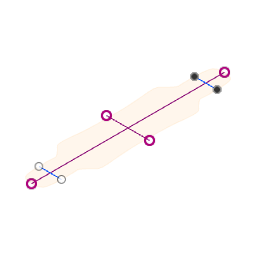
LongBoard v1 (Autodesk Fusion 360 design; units mm, degrees)
Autodesk Fusion 360 part; units mm, degrees
sketch "Sketch1" plane through (0, 0, 0) normal (0, 1, 0) x (1, 0, 0)
  line L0 (1.5, -63) -> (1.5, 40)
  line L1 (-10, -11.5) -> (13, -11.5)
  spline S0 degree 5 poles (1.5, 39.8994) (1.4399, 39.8994) (1.3198, 39.8994) (1.1397, 39.8994) (0.8995, 39.8994) (0.5992, 39.8994) (0.359, 39.8994) (0.1788, 39.8994) (0.0587, 39.8994) (-0.0013, 39.8994) knots 0 0 0 0 0 0 0.2 0.4 0.6 0.8 1 1 1 1 1 1
  spline S1 degree 5 poles (-0.0013, 39.8994) (-0.0218, 39.8979) (-0.0631, 39.8948) (-0.1256, 39.8901) (-0.2101, 39.8836) (-0.3178, 39.8751) (-0.4274, 39.866) (-0.539, 39.8561) (-0.6523, 39.8451) (-0.7672, 39.8322) (-0.8833, 39.8166) (-1.0002, 39.7977) (-1.1173, 39.7746) (-1.2334, 39.7472) (-1.3473, 39.7155) (-1.457, 39.6802) (-1.5606, 39.6428) (-1.6561, 39.6046) (-1.7423, 39.5672) (-1.8188, 39.5315) (-1.887, 39.4978) (-1.9498, 39.4653) (-2.0108, 39.4326) (-2.0739, 39.398) (-2.1421, 39.3599) (-2.2168, 39.3165) (-2.2984, 39.2666) (-2.3861, 39.2095) (-2.4785, 39.1451) (-2.5733, 39.074) (-2.6681, 38.9982) (-2.7601, 38.9197) (-2.847, 38.8412) (-2.9267, 38.765) (-2.9978, 38.693) (-3.0602, 38.6264) (-3.1145, 38.5652) (-3.1625, 38.5087) (-3.2058, 38.4556) (-3.2464, 38.4044) (-3.2854, 38.3535) (-3.3238, 38.3017) (-3.3617, 38.2481) (-3.399, 38.1932) (-3.4348, 38.1384) (-3.4682, 38.0857) (-3.4986, 38.0364) (-3.526, 37.9902) (-3.5515, 37.9451) (-3.5761, 37.8985) (-3.6006, 37.849) (-3.6247, 37.7981) (-3.6475, 37.7483) (-3.6682, 37.7019) (-3.6867, 37.6585) (-3.7041, 37.6146) (-3.7216, 37.5664) (-3.7401, 37.5116) (-3.7593, 37.4514) (-3.7786, 37.3886) (-3.7971, 37.3266) (-3.8143, 37.2668) (-3.8302, 37.2087) (-3.8451, 37.1506) (-3.8597, 37.0905) (-3.8743, 37.0273) (-3.8893, 36.9608) (-3.9052, 36.8908) (-3.922, 36.8176) (-3.9395, 36.7407) (-3.9576, 36.6596) (-3.9757, 36.5739) (-3.9934, 36.4839) (-4.0103, 36.3909) (-4.0261, 36.2973) (-4.0406, 36.2061) (-4.0536, 36.1202) (-4.0654, 36.0413) (-4.0759, 35.9695) (-4.0855, 35.9031) (-4.0946, 35.8392) (-4.1035, 35.775) (-4.1124, 35.7085) (-4.1217, 35.639) (-4.1314, 35.5666) (-4.1416, 35.4919) (-4.152, 35.4162) (-4.1625, 35.3404) (-4.1727, 35.2657) (-4.1824, 35.1926) (-4.1915, 35.1209) (-4.2002, 35.0493) (-4.2087, 34.9764) (-4.2174, 34.9005) (-4.2265, 34.8206) (-4.2359, 34.7364) (-4.2456, 34.6486) (-4.2552, 34.5584) (-4.2646, 34.4672) (-4.2736, 34.3769) (-4.2821, 34.2889) (-4.2901, 34.2046) (-4.2977, 34.1248) (-4.3048, 34.0496) (-4.3115, 33.9782) (-4.318, 33.9088) (-4.3244, 33.8391) (-4.3307, 33.7658) (-4.3372, 33.6856) (-4.3442, 33.5945) (-4.3518, 33.4891) (-4.3603, 33.3661) (-4.3699, 33.2229) (-4.3806, 33.0582) (-4.3925, 32.8718) (-4.4053, 32.6647) (-4.4189, 32.4387) (-4.433, 32.1966) (-4.4474, 31.9415) (-4.4617, 31.677) (-4.4756, 31.4069) (-4.4888, 31.1352) (-4.5011, 30.8654) (-4.5122, 30.6012) (-4.522, 30.3455) (-4.5305, 30.1006) (-4.5377, 29.8683) (-4.5436, 29.6498) (-4.5484, 29.4457) (-4.5522, 29.2561) (-4.5552, 29.0807) (-4.5576, 28.9186) (-4.5595, 28.7685) (-4.5611, 28.6286) (-4.5624, 28.4967) (-4.5636, 28.3702) (-4.5646, 28.2466) (-4.5654, 28.1229) (-4.5661, 27.9966) (-4.5666, 27.8653) (-4.5669, 27.7268) (-4.567, 27.5796) (-4.5669, 27.4226) (-4.5665, 27.2548) (-4.5659, 27.0757) (-4.5651, 26.8851) (-4.5642, 26.7231) (-4.5634, 26.5963) (-4.5628, 26.5094) (-4.5625, 26.4653) knots 0 0 0 0 0 0 0.00689655 0.0137931 0.02068966 0.02758621 0.03448276 0.04137931 0.04827586 0.05517241 0.06206897 0.06896552 0.07586207 0.08275862 0.08965517 0.09655172 0.10344828 0.11034483 0.11724138 0.12413793 0.13103448 0.13793103 0.14482759 0.15172414 0.15862069 0.16551724 0.17241379 0.17931034 0.1862069 0.19310345 0.2 0.20689655 0.2137931 0.22068966 0.22758621 0.23448276 0.24137931 0.24827586 0.25517241 0.26206897 0.26896552 0.27586207 0.28275862 0.28965517 0.29655172 0.30344828 0.31034483 0.31724138 0.32413793 0.33103448 0.33793103 0.34482759 0.35172414 0.35862069 0.36551724 0.37241379 0.37931034 0.3862069 0.39310345 0.4 0.40689655 0.4137931 0.42068966 0.42758621 0.43448276 0.44137931 0.44827586 0.45517241 0.46206897 0.46896552 0.47586207 0.48275862 0.48965517 0.49655172 0.50344828 0.51034483 0.51724138 0.52413793 0.53103448 0.53793103 0.54482759 0.55172414 0.55862069 0.56551724 0.57241379 0.57931034 0.5862069 0.59310345 0.6 0.60689655 0.6137931 0.62068966 0.62758621 0.63448276 0.64137931 0.64827586 0.65517241 0.66206897 0.66896552 0.67586207 0.68275862 0.68965517 0.69655172 0.70344828 0.71034483 0.71724138 0.72413793 0.73103448 0.73793103 0.74482759 0.75172414 0.75862069 0.76551724 0.77241379 0.77931034 0.7862069 0.79310345 0.8 0.80689655 0.8137931 0.82068966 0.82758621 0.83448276 0.84137931 0.84827586 0.85517241 0.86206897 0.86896552 0.87586207 0.88275862 0.88965517 0.89655172 0.90344828 0.91034483 0.91724138 0.92413793 0.93103448 0.93793103 0.94482759 0.95172414 0.95862069 0.96551724 0.97241379 0.97931034 0.9862069 0.99310345 1 1 1 1 1 1
  spline S2 degree 5 poles (-4.5625, 26.4653) (-4.5655, 26.3307) (-4.57, 26.0496) (-4.572, 25.5928) (-4.5661, 24.9124) (-4.5379, 23.9635) (-4.4825, 22.9635) (-4.3594, 22.0422) (-4.344, 21.226) (-4.6467, 20.4795) (-5.3052, 19.6439) (-6.1392, 18.6182) (-7.0385, 17.5852) (-7.8877, 16.7191) (-8.6091, 16.1406) (-9.1643, 15.5973) (-9.5444, 14.8768) (-9.7555, 13.8923) (-9.8172, 12.6021) (-9.7558, 10.9978) (-9.602, 9.0799) (-9.389, 6.8619) (-9.151, 4.3636) (-8.9215, 1.6101) (-8.732, -1.3722) (-8.61, -4.5579) (-8.5838, -7.2519) (-8.6109, -9.3475) (-8.6505, -10.7771) (-8.6757, -11.5) knots 0 0 0 0 0 0 0.04 0.08 0.12 0.16 0.2 0.24 0.28 0.32 0.36 0.4 0.44 0.48 0.52 0.56 0.6 0.64 0.68 0.72 0.76 0.8 0.84 0.88 0.92 0.96 1 1 1 1 1 1
  line L2 (-5.8, 18.6) -> (-11, 14)
  line L3 (-2.8, 23.5) -> (-6.8, 17.2)
  line L4 (-4.8152, 28.0337) -> (-4.1848, 18.7663)
  line L5 (-8.4763, -5.7777) -> (-8.8751, -17.2223)
  spline S3 degree 5 poles (-4.5625, -49.4653) (-4.5655, -49.3307) (-4.57, -49.0496) (-4.572, -48.5928) (-4.5661, -47.9124) (-4.5379, -46.9635) (-4.4825, -45.9635) (-4.3594, -45.0422) (-4.344, -44.226) (-4.6467, -43.4795) (-5.3052, -42.6439) (-6.1392, -41.6182) (-7.0385, -40.5852) (-7.8877, -39.7191) (-8.6091, -39.1406) (-9.1643, -38.5973) (-9.5444, -37.8768) (-9.7555, -36.8923) (-9.8172, -35.6021) (-9.7558, -33.9978) (-9.602, -32.0799) (-9.389, -29.8619) (-9.151, -27.3636) (-8.9215, -24.6101) (-8.732, -21.6278) (-8.61, -18.4421) (-8.5838, -15.7481) (-8.6109, -13.6525) (-8.6505, -12.2229) (-8.6757, -11.5) knots 0 0 0 0 0 0 0.04 0.08 0.12 0.16 0.2 0.24 0.28 0.32 0.36 0.4 0.44 0.48 0.52 0.56 0.6 0.64 0.68 0.72 0.76 0.8 0.84 0.88 0.92 0.96 1 1 1 1 1 1
  line L6 (-4.4911, 29.6841) -> (-4.634, 23.2466)
  line L7 (-4.4911, -52.6841) -> (-4.634, -46.2466)
  line L8 (-4.8152, -51.0337) -> (-4.1848, -41.7663)
  line L9 (-2.8, -46.5) -> (-6.8, -40.2)
  line L10 (-5.8, -41.6) -> (-11, -37)
  line L11 (-8.4763, -17.2223) -> (-8.8751, -5.7777)
  spline S4 degree 5 poles (-0.0013, -62.8994) (-0.0218, -62.8979) (-0.0631, -62.8948) (-0.1256, -62.8901) (-0.2101, -62.8836) (-0.3178, -62.8751) (-0.4274, -62.866) (-0.539, -62.8561) (-0.6523, -62.8451) (-0.7672, -62.8322) (-0.8833, -62.8166) (-1.0002, -62.7977) (-1.1173, -62.7746) (-1.2334, -62.7472) (-1.3473, -62.7155) (-1.457, -62.6802) (-1.5606, -62.6428) (-1.6561, -62.6046) (-1.7423, -62.5672) (-1.8188, -62.5315) (-1.887, -62.4978) (-1.9498, -62.4653) (-2.0108, -62.4326) (-2.0739, -62.398) (-2.1421, -62.3599) (-2.2168, -62.3165) (-2.2984, -62.2666) (-2.3861, -62.2095) (-2.4785, -62.1451) (-2.5733, -62.074) (-2.6681, -61.9982) (-2.7601, -61.9197) (-2.847, -61.8412) (-2.9267, -61.765) (-2.9978, -61.693) (-3.0602, -61.6264) (-3.1145, -61.5652) (-3.1625, -61.5087) (-3.2058, -61.4556) (-3.2464, -61.4044) (-3.2854, -61.3535) (-3.3238, -61.3017) (-3.3617, -61.2481) (-3.399, -61.1932) (-3.4348, -61.1384) (-3.4682, -61.0857) (-3.4986, -61.0364) (-3.526, -60.9902) (-3.5515, -60.9451) (-3.5761, -60.8985) (-3.6006, -60.849) (-3.6247, -60.7981) (-3.6475, -60.7483) (-3.6682, -60.7019) (-3.6867, -60.6585) (-3.7041, -60.6146) (-3.7216, -60.5664) (-3.7401, -60.5116) (-3.7593, -60.4514) (-3.7786, -60.3886) (-3.7971, -60.3266) (-3.8143, -60.2668) (-3.8302, -60.2087) (-3.8451, -60.1506) (-3.8597, -60.0905) (-3.8743, -60.0273) (-3.8893, -59.9608) (-3.9052, -59.8908) (-3.922, -59.8176) (-3.9395, -59.7407) (-3.9576, -59.6596) (-3.9757, -59.5739) (-3.9934, -59.4839) (-4.0103, -59.3909) (-4.0261, -59.2973) (-4.0406, -59.2061) (-4.0536, -59.1202) (-4.0654, -59.0413) (-4.0759, -58.9695) (-4.0855, -58.9031) (-4.0946, -58.8392) (-4.1035, -58.775) (-4.1124, -58.7085) (-4.1217, -58.639) (-4.1314, -58.5666) (-4.1416, -58.4919) (-4.152, -58.4162) (-4.1625, -58.3404) (-4.1727, -58.2657) (-4.1824, -58.1926) (-4.1915, -58.1209) (-4.2002, -58.0493) (-4.2087, -57.9764) (-4.2174, -57.9005) (-4.2265, -57.8206) (-4.2359, -57.7364) (-4.2456, -57.6486) (-4.2552, -57.5584) (-4.2646, -57.4672) (-4.2736, -57.3769) (-4.2821, -57.2889) (-4.2901, -57.2046) (-4.2977, -57.1248) (-4.3048, -57.0496) (-4.3115, -56.9782) (-4.318, -56.9088) (-4.3244, -56.8391) (-4.3307, -56.7658) (-4.3372, -56.6856) (-4.3442, -56.5945) (-4.3518, -56.4891) (-4.3603, -56.3661) (-4.3699, -56.2229) (-4.3806, -56.0582) (-4.3925, -55.8718) (-4.4053, -55.6647) (-4.4189, -55.4387) (-4.433, -55.1966) (-4.4474, -54.9415) (-4.4617, -54.677) (-4.4756, -54.4069) (-4.4888, -54.1352) (-4.5011, -53.8654) (-4.5122, -53.6012) (-4.522, -53.3455) (-4.5305, -53.1006) (-4.5377, -52.8683) (-4.5436, -52.6498) (-4.5484, -52.4457) (-4.5522, -52.2561) (-4.5552, -52.0807) (-4.5576, -51.9186) (-4.5595, -51.7685) (-4.5611, -51.6286) (-4.5624, -51.4967) (-4.5636, -51.3702) (-4.5646, -51.2466) (-4.5654, -51.1229) (-4.5661, -50.9966) (-4.5666, -50.8653) (-4.5669, -50.7268) (-4.567, -50.5796) (-4.5669, -50.4226) (-4.5665, -50.2548) (-4.5659, -50.0757) (-4.5651, -49.8851) (-4.5642, -49.7231) (-4.5634, -49.5963) (-4.5628, -49.5094) (-4.5625, -49.4653) knots 0 0 0 0 0 0 0.00689655 0.0137931 0.02068966 0.02758621 0.03448276 0.04137931 0.04827586 0.05517241 0.06206897 0.06896552 0.07586207 0.08275862 0.08965517 0.09655172 0.10344828 0.11034483 0.11724138 0.12413793 0.13103448 0.13793103 0.14482759 0.15172414 0.15862069 0.16551724 0.17241379 0.17931034 0.1862069 0.19310345 0.2 0.20689655 0.2137931 0.22068966 0.22758621 0.23448276 0.24137931 0.24827586 0.25517241 0.26206897 0.26896552 0.27586207 0.28275862 0.28965517 0.29655172 0.30344828 0.31034483 0.31724138 0.32413793 0.33103448 0.33793103 0.34482759 0.35172414 0.35862069 0.36551724 0.37241379 0.37931034 0.3862069 0.39310345 0.4 0.40689655 0.4137931 0.42068966 0.42758621 0.43448276 0.44137931 0.44827586 0.45517241 0.46206897 0.46896552 0.47586207 0.48275862 0.48965517 0.49655172 0.50344828 0.51034483 0.51724138 0.52413793 0.53103448 0.53793103 0.54482759 0.55172414 0.55862069 0.56551724 0.57241379 0.57931034 0.5862069 0.59310345 0.6 0.60689655 0.6137931 0.62068966 0.62758621 0.63448276 0.64137931 0.64827586 0.65517241 0.66206897 0.66896552 0.67586207 0.68275862 0.68965517 0.69655172 0.70344828 0.71034483 0.71724138 0.72413793 0.73103448 0.73793103 0.74482759 0.75172414 0.75862069 0.76551724 0.77241379 0.77931034 0.7862069 0.79310345 0.8 0.80689655 0.8137931 0.82068966 0.82758621 0.83448276 0.84137931 0.84827586 0.85517241 0.86206897 0.86896552 0.87586207 0.88275862 0.88965517 0.89655172 0.90344828 0.91034483 0.91724138 0.92413793 0.93103448 0.93793103 0.94482759 0.95172414 0.95862069 0.96551724 0.97241379 0.97931034 0.9862069 0.99310345 1 1 1 1 1 1
  line L12 (1.5328, 40.0122) -> (-1.5354, 39.7866)
  line L13 (-4.5763, 28.5249) -> (-4.5488, 24.4057)
  line L14 (1.5328, -63.0122) -> (-1.5354, -62.7866)
  line L15 (-4.5763, -51.5249) -> (-4.5488, -47.4057)
  spline S5 degree 5 poles (1.5, -62.8994) (1.4399, -62.8994) (1.3198, -62.8994) (1.1397, -62.8994) (0.8995, -62.8994) (0.5992, -62.8994) (0.359, -62.8994) (0.1788, -62.8994) (0.0587, -62.8994) (-0.0013, -62.8994) knots 0 0 0 0 0 0 0.2 0.4 0.6 0.8 1 1 1 1 1 1
  line L16 (1.6531, 39.8994) -> (1.3469, 39.8994)
  line L17 (0.1518, 39.8994) -> (-0.1544, 39.8994)
  line L18 (1.6531, -62.8994) -> (1.3469, -62.8994)
  line L19 (0.1518, -62.8994) -> (-0.1544, -62.8994)
  spline S6 degree 5 poles (7.5625, 26.4653) (7.5655, 26.3307) (7.57, 26.0496) (7.572, 25.5928) (7.5661, 24.9124) (7.5379, 23.9635) (7.4825, 22.9635) (7.3594, 22.0422) (7.344, 21.226) (7.6467, 20.4795) (8.3052, 19.6439) (9.1392, 18.6182) (10.0385, 17.5852) (10.8877, 16.7191) (11.6091, 16.1406) (12.1643, 15.5973) (12.5444, 14.8768) (12.7555, 13.8923) (12.8172, 12.6021) (12.7558, 10.9978) (12.602, 9.0799) (12.389, 6.8619) (12.151, 4.3636) (11.9215, 1.6101) (11.732, -1.3722) (11.61, -4.5579) (11.5838, -7.2519) (11.6109, -9.3475) (11.6505, -10.7771) (11.6757, -11.5) knots 0 0 0 0 0 0 0.04 0.08 0.12 0.16 0.2 0.24 0.28 0.32 0.36 0.4 0.44 0.48 0.52 0.56 0.6 0.64 0.68 0.72 0.76 0.8 0.84 0.88 0.92 0.96 1 1 1 1 1 1
  line L20 (7.4911, 29.6841) -> (7.634, 23.2466)
  line L21 (7.8152, 28.0337) -> (7.1848, 18.7663)
  line L22 (5.8, 23.5) -> (9.8, 17.2)
  line L23 (8.8, 18.6) -> (14, 14)
  line L24 (11.4763, -5.7777) -> (11.8751, -17.2223)
  spline S7 degree 5 poles (7.5625, -49.4653) (7.5655, -49.3307) (7.57, -49.0496) (7.572, -48.5928) (7.5661, -47.9124) (7.5379, -46.9635) (7.4825, -45.9635) (7.3594, -45.0422) (7.344, -44.226) (7.6467, -43.4795) (8.3052, -42.6439) (9.1392, -41.6182) (10.0385, -40.5852) (10.8877, -39.7191) (11.6091, -39.1406) (12.1643, -38.5973) (12.5444, -37.8768) (12.7555, -36.8923) (12.8172, -35.6021) (12.7558, -33.9978) (12.602, -32.0799) (12.389, -29.8619) (12.151, -27.3636) (11.9215, -24.6101) (11.732, -21.6278) (11.61, -18.4421) (11.5838, -15.7481) (11.6109, -13.6525) (11.6505, -12.2229) (11.6757, -11.5) knots 0 0 0 0 0 0 0.04 0.08 0.12 0.16 0.2 0.24 0.28 0.32 0.36 0.4 0.44 0.48 0.52 0.56 0.6 0.64 0.68 0.72 0.76 0.8 0.84 0.88 0.92 0.96 1 1 1 1 1 1
  line L25 (7.4911, -52.6841) -> (7.634, -46.2466)
  line L26 (7.8152, -51.0337) -> (7.1848, -41.7663)
  line L27 (5.8, -46.5) -> (9.8, -40.2)
  line L28 (8.8, -41.6) -> (14, -37)
  line L29 (11.4763, -17.2223) -> (11.8751, -5.7777)
  spline S8 degree 5 poles (3.0013, 39.8994) (3.0218, 39.8979) (3.0631, 39.8948) (3.1256, 39.8901) (3.2101, 39.8836) (3.3178, 39.8751) (3.4274, 39.866) (3.539, 39.8561) (3.6523, 39.8451) (3.7672, 39.8322) (3.8833, 39.8166) (4.0002, 39.7977) (4.1173, 39.7746) (4.2334, 39.7472) (4.3473, 39.7155) (4.457, 39.6802) (4.5606, 39.6428) (4.6561, 39.6046) (4.7423, 39.5672) (4.8188, 39.5315) (4.887, 39.4978) (4.9498, 39.4653) (5.0108, 39.4326) (5.0739, 39.398) (5.1421, 39.3599) (5.2168, 39.3165) (5.2984, 39.2666) (5.3861, 39.2095) (5.4785, 39.1451) (5.5733, 39.074) (5.6681, 38.9982) (5.7601, 38.9197) (5.847, 38.8412) (5.9267, 38.765) (5.9978, 38.693) (6.0602, 38.6264) (6.1145, 38.5652) (6.1625, 38.5087) (6.2058, 38.4556) (6.2464, 38.4044) (6.2854, 38.3535) (6.3238, 38.3017) (6.3617, 38.2481) (6.399, 38.1932) (6.4348, 38.1384) (6.4682, 38.0857) (6.4986, 38.0364) (6.526, 37.9902) (6.5515, 37.9451) (6.5761, 37.8985) (6.6006, 37.849) (6.6247, 37.7981) (6.6475, 37.7483) (6.6682, 37.7019) (6.6867, 37.6585) (6.7041, 37.6146) (6.7216, 37.5664) (6.7401, 37.5116) (6.7593, 37.4514) (6.7786, 37.3886) (6.7971, 37.3266) (6.8143, 37.2668) (6.8302, 37.2087) (6.8451, 37.1506) (6.8597, 37.0905) (6.8743, 37.0273) (6.8893, 36.9608) (6.9052, 36.8908) (6.922, 36.8176) (6.9395, 36.7407) (6.9576, 36.6596) (6.9757, 36.5739) (6.9934, 36.4839) (7.0103, 36.3909) (7.0261, 36.2973) (7.0406, 36.2061) (7.0536, 36.1202) (7.0654, 36.0413) (7.0759, 35.9695) (7.0855, 35.9031) (7.0946, 35.8392) (7.1035, 35.775) (7.1124, 35.7085) (7.1217, 35.639) (7.1314, 35.5666) (7.1416, 35.4919) (7.152, 35.4162) (7.1625, 35.3404) (7.1727, 35.2657) (7.1824, 35.1926) (7.1915, 35.1209) (7.2002, 35.0493) (7.2087, 34.9764) (7.2174, 34.9005) (7.2265, 34.8206) (7.2359, 34.7364) (7.2456, 34.6486) (7.2552, 34.5584) (7.2646, 34.4672) (7.2736, 34.3769) (7.2821, 34.2889) (7.2901, 34.2046) (7.2977, 34.1248) (7.3048, 34.0496) (7.3115, 33.9782) (7.318, 33.9088) (7.3244, 33.8391) (7.3307, 33.7658) (7.3372, 33.6856) (7.3442, 33.5945) (7.3518, 33.4891) (7.3603, 33.3661) (7.3699, 33.2229) (7.3806, 33.0582) (7.3925, 32.8718) (7.4053, 32.6647) (7.4189, 32.4387) (7.433, 32.1966) (7.4474, 31.9415) (7.4617, 31.677) (7.4756, 31.4069) (7.4888, 31.1352) (7.5011, 30.8654) (7.5122, 30.6012) (7.522, 30.3455) (7.5305, 30.1006) (7.5377, 29.8683) (7.5436, 29.6498) (7.5484, 29.4457) (7.5522, 29.2561) (7.5552, 29.0807) (7.5576, 28.9186) (7.5595, 28.7685) (7.5611, 28.6286) (7.5624, 28.4967) (7.5636, 28.3702) (7.5646, 28.2466) (7.5654, 28.1229) (7.5661, 27.9966) (7.5666, 27.8653) (7.5669, 27.7268) (7.567, 27.5796) (7.5669, 27.4226) (7.5665, 27.2548) (7.5659, 27.0757) (7.5651, 26.8851) (7.5642, 26.7231) (7.5634, 26.5963) (7.5628, 26.5094) (7.5625, 26.4653) knots 0 0 0 0 0 0 0.00689655 0.0137931 0.02068966 0.02758621 0.03448276 0.04137931 0.04827586 0.05517241 0.06206897 0.06896552 0.07586207 0.08275862 0.08965517 0.09655172 0.10344828 0.11034483 0.11724138 0.12413793 0.13103448 0.13793103 0.14482759 0.15172414 0.15862069 0.16551724 0.17241379 0.17931034 0.1862069 0.19310345 0.2 0.20689655 0.2137931 0.22068966 0.22758621 0.23448276 0.24137931 0.24827586 0.25517241 0.26206897 0.26896552 0.27586207 0.28275862 0.28965517 0.29655172 0.30344828 0.31034483 0.31724138 0.32413793 0.33103448 0.33793103 0.34482759 0.35172414 0.35862069 0.36551724 0.37241379 0.37931034 0.3862069 0.39310345 0.4 0.40689655 0.4137931 0.42068966 0.42758621 0.43448276 0.44137931 0.44827586 0.45517241 0.46206897 0.46896552 0.47586207 0.48275862 0.48965517 0.49655172 0.50344828 0.51034483 0.51724138 0.52413793 0.53103448 0.53793103 0.54482759 0.55172414 0.55862069 0.56551724 0.57241379 0.57931034 0.5862069 0.59310345 0.6 0.60689655 0.6137931 0.62068966 0.62758621 0.63448276 0.64137931 0.64827586 0.65517241 0.66206897 0.66896552 0.67586207 0.68275862 0.68965517 0.69655172 0.70344828 0.71034483 0.71724138 0.72413793 0.73103448 0.73793103 0.74482759 0.75172414 0.75862069 0.76551724 0.77241379 0.77931034 0.7862069 0.79310345 0.8 0.80689655 0.8137931 0.82068966 0.82758621 0.83448276 0.84137931 0.84827586 0.85517241 0.86206897 0.86896552 0.87586207 0.88275862 0.88965517 0.89655172 0.90344828 0.91034483 0.91724138 0.92413793 0.93103448 0.93793103 0.94482759 0.95172414 0.95862069 0.96551724 0.97241379 0.97931034 0.9862069 0.99310345 1 1 1 1 1 1
  line L30 (1.4672, 40.0122) -> (4.5354, 39.7866)
  line L31 (7.5763, 28.5249) -> (7.5488, 24.4057)
  spline S9 degree 5 poles (1.5, 39.8994) (1.5601, 39.8994) (1.6802, 39.8994) (1.8603, 39.8994) (2.1005, 39.8994) (2.4008, 39.8994) (2.641, 39.8994) (2.8212, 39.8994) (2.9413, 39.8994) (3.0013, 39.8994) knots 0 0 0 0 0 0 0.2 0.4 0.6 0.8 1 1 1 1 1 1
  line L32 (1.3469, 39.8994) -> (1.6531, 39.8994)
  line L33 (2.8482, 39.8994) -> (3.1544, 39.8994)
  spline S10 degree 5 poles (3.0013, -62.8994) (3.0218, -62.8979) (3.0631, -62.8948) (3.1256, -62.8901) (3.2101, -62.8836) (3.3178, -62.8751) (3.4274, -62.866) (3.539, -62.8561) (3.6523, -62.8451) (3.7672, -62.8322) (3.8833, -62.8166) (4.0002, -62.7977) (4.1173, -62.7746) (4.2334, -62.7472) (4.3473, -62.7155) (4.457, -62.6802) (4.5606, -62.6428) (4.6561, -62.6046) (4.7423, -62.5672) (4.8188, -62.5315) (4.887, -62.4978) (4.9498, -62.4653) (5.0108, -62.4326) (5.0739, -62.398) (5.1421, -62.3599) (5.2168, -62.3165) (5.2984, -62.2666) (5.3861, -62.2095) (5.4785, -62.1451) (5.5733, -62.074) (5.6681, -61.9982) (5.7601, -61.9197) (5.847, -61.8412) (5.9267, -61.765) (5.9978, -61.693) (6.0602, -61.6264) (6.1145, -61.5652) (6.1625, -61.5087) (6.2058, -61.4556) (6.2464, -61.4044) (6.2854, -61.3535) (6.3238, -61.3017) (6.3617, -61.2481) (6.399, -61.1932) (6.4348, -61.1384) (6.4682, -61.0857) (6.4986, -61.0364) (6.526, -60.9902) (6.5515, -60.9451) (6.5761, -60.8985) (6.6006, -60.849) (6.6247, -60.7981) (6.6475, -60.7483) (6.6682, -60.7019) (6.6867, -60.6585) (6.7041, -60.6146) (6.7216, -60.5664) (6.7401, -60.5116) (6.7593, -60.4514) (6.7786, -60.3886) (6.7971, -60.3266) (6.8143, -60.2668) (6.8302, -60.2087) (6.8451, -60.1506) (6.8597, -60.0905) (6.8743, -60.0273) (6.8893, -59.9608) (6.9052, -59.8908) (6.922, -59.8176) (6.9395, -59.7407) (6.9576, -59.6596) (6.9757, -59.5739) (6.9934, -59.4839) (7.0103, -59.3909) (7.0261, -59.2973) (7.0406, -59.2061) (7.0536, -59.1202) (7.0654, -59.0413) (7.0759, -58.9695) (7.0855, -58.9031) (7.0946, -58.8392) (7.1035, -58.775) (7.1124, -58.7085) (7.1217, -58.639) (7.1314, -58.5666) (7.1416, -58.4919) (7.152, -58.4162) (7.1625, -58.3404) (7.1727, -58.2657) (7.1824, -58.1926) (7.1915, -58.1209) (7.2002, -58.0493) (7.2087, -57.9764) (7.2174, -57.9005) (7.2265, -57.8206) (7.2359, -57.7364) (7.2456, -57.6486) (7.2552, -57.5584) (7.2646, -57.4672) (7.2736, -57.3769) (7.2821, -57.2889) (7.2901, -57.2046) (7.2977, -57.1248) (7.3048, -57.0496) (7.3115, -56.9782) (7.318, -56.9088) (7.3244, -56.8391) (7.3307, -56.7658) (7.3372, -56.6856) (7.3442, -56.5945) (7.3518, -56.4891) (7.3603, -56.3661) (7.3699, -56.2229) (7.3806, -56.0582) (7.3925, -55.8718) (7.4053, -55.6647) (7.4189, -55.4387) (7.433, -55.1966) (7.4474, -54.9415) (7.4617, -54.677) (7.4756, -54.4069) (7.4888, -54.1352) (7.5011, -53.8654) (7.5122, -53.6012) (7.522, -53.3455) (7.5305, -53.1006) (7.5377, -52.8683) (7.5436, -52.6498) (7.5484, -52.4457) (7.5522, -52.2561) (7.5552, -52.0807) (7.5576, -51.9186) (7.5595, -51.7685) (7.5611, -51.6286) (7.5624, -51.4967) (7.5636, -51.3702) (7.5646, -51.2466) (7.5654, -51.1229) (7.5661, -50.9966) (7.5666, -50.8653) (7.5669, -50.7268) (7.567, -50.5796) (7.5669, -50.4226) (7.5665, -50.2548) (7.5659, -50.0757) (7.5651, -49.8851) (7.5642, -49.7231) (7.5634, -49.5963) (7.5628, -49.5094) (7.5625, -49.4653) knots 0 0 0 0 0 0 0.00689655 0.0137931 0.02068966 0.02758621 0.03448276 0.04137931 0.04827586 0.05517241 0.06206897 0.06896552 0.07586207 0.08275862 0.08965517 0.09655172 0.10344828 0.11034483 0.11724138 0.12413793 0.13103448 0.13793103 0.14482759 0.15172414 0.15862069 0.16551724 0.17241379 0.17931034 0.1862069 0.19310345 0.2 0.20689655 0.2137931 0.22068966 0.22758621 0.23448276 0.24137931 0.24827586 0.25517241 0.26206897 0.26896552 0.27586207 0.28275862 0.28965517 0.29655172 0.30344828 0.31034483 0.31724138 0.32413793 0.33103448 0.33793103 0.34482759 0.35172414 0.35862069 0.36551724 0.37241379 0.37931034 0.3862069 0.39310345 0.4 0.40689655 0.4137931 0.42068966 0.42758621 0.43448276 0.44137931 0.44827586 0.45517241 0.46206897 0.46896552 0.47586207 0.48275862 0.48965517 0.49655172 0.50344828 0.51034483 0.51724138 0.52413793 0.53103448 0.53793103 0.54482759 0.55172414 0.55862069 0.56551724 0.57241379 0.57931034 0.5862069 0.59310345 0.6 0.60689655 0.6137931 0.62068966 0.62758621 0.63448276 0.64137931 0.64827586 0.65517241 0.66206897 0.66896552 0.67586207 0.68275862 0.68965517 0.69655172 0.70344828 0.71034483 0.71724138 0.72413793 0.73103448 0.73793103 0.74482759 0.75172414 0.75862069 0.76551724 0.77241379 0.77931034 0.7862069 0.79310345 0.8 0.80689655 0.8137931 0.82068966 0.82758621 0.83448276 0.84137931 0.84827586 0.85517241 0.86206897 0.86896552 0.87586207 0.88275862 0.88965517 0.89655172 0.90344828 0.91034483 0.91724138 0.92413793 0.93103448 0.93793103 0.94482759 0.95172414 0.95862069 0.96551724 0.97241379 0.97931034 0.9862069 0.99310345 1 1 1 1 1 1
  line L34 (1.4672, -63.0122) -> (4.5354, -62.7866)
  line L35 (7.5763, -51.5249) -> (7.5488, -47.4057)
  spline S11 degree 5 poles (1.5, -62.8994) (1.5601, -62.8994) (1.6802, -62.8994) (1.8603, -62.8994) (2.1005, -62.8994) (2.4008, -62.8994) (2.641, -62.8994) (2.8212, -62.8994) (2.9413, -62.8994) (3.0013, -62.8994) knots 0 0 0 0 0 0 0.2 0.4 0.6 0.8 1 1 1 1 1 1
  line L36 (1.3469, -62.8994) -> (1.6531, -62.8994)
  line L37 (2.8482, -62.8994) -> (3.1544, -62.8994)
  point P0 (-2262.415, 0)
  point P1 (-2262.415, 0)
extrude "Extrude1" add sketch "Sketch1" along normal blind 1 contours L0 L1 S3 L8 L9 L10 S4 L15 S5 L18 L19 L36 | L0 L1 L18 S7 L26 L27 S10 L35 S11 L36 L37 | L0 L1 S0 S1 S2 L3 L4 L13 L16 L17 L32 | L0 L1 L16 S6 L21 L22 L23 S8 L31 S9 L32 L33 | S3 L9 L10 | S6 L22 L23 | S2 L3 L4 | S3 L8 L9 | S6 L21 L22 | S7 L26 L27
sketch "Sketch2" plane through (0, 1, 0) normal (0, 1, 0) x (-1, 0, 0)
  line L0 (0.0013, 62.8994) -> (-1.5, 62.8994)
  line L1 (-1.5, 62.8994) -> (-3.0013, 62.8994)
  spline S0 degree 5 poles (-3.0013, 62.8994) (-3.0218, 62.8979) (-3.0631, 62.8948) (-3.1256, 62.8901) (-3.2101, 62.8836) (-3.3178, 62.8751) (-3.4274, 62.866) (-3.539, 62.8561) (-3.6523, 62.8451) (-3.7672, 62.8322) (-3.8833, 62.8166) (-4.0002, 62.7977) (-4.1173, 62.7746) (-4.2334, 62.7472) (-4.3473, 62.7155) (-4.457, 62.6802) (-4.5606, 62.6428) (-4.6561, 62.6046) (-4.7423, 62.5672) (-4.8188, 62.5315) (-4.887, 62.4978) (-4.9498, 62.4653) (-5.0108, 62.4326) (-5.0739, 62.398) (-5.1421, 62.3599) (-5.2168, 62.3165) (-5.2984, 62.2666) (-5.3861, 62.2095) (-5.4785, 62.1451) (-5.5733, 62.074) (-5.6681, 61.9982) (-5.7601, 61.9197) (-5.847, 61.8412) (-5.9267, 61.765) (-5.9978, 61.693) (-6.0602, 61.6264) (-6.1145, 61.5652) (-6.1625, 61.5087) (-6.2058, 61.4556) (-6.2464, 61.4044) (-6.2854, 61.3535) (-6.3238, 61.3017) (-6.3617, 61.2481) (-6.399, 61.1932) (-6.4348, 61.1384) (-6.4682, 61.0857) (-6.4986, 61.0364) (-6.526, 60.9902) (-6.5515, 60.9451) (-6.5761, 60.8985) (-6.6006, 60.849) (-6.6247, 60.7981) (-6.6475, 60.7483) (-6.6682, 60.7019) (-6.6867, 60.6585) (-6.7041, 60.6146) (-6.7216, 60.5664) (-6.7401, 60.5116) (-6.7593, 60.4514) (-6.7786, 60.3886) (-6.7971, 60.3266) (-6.8143, 60.2668) (-6.8302, 60.2087) (-6.8451, 60.1506) (-6.8597, 60.0905) (-6.8743, 60.0273) (-6.8893, 59.9608) (-6.9052, 59.8908) (-6.922, 59.8176) (-6.9395, 59.7407) (-6.9576, 59.6596) (-6.9757, 59.5739) (-6.9934, 59.4839) (-7.0103, 59.3909) (-7.0261, 59.2973) (-7.0406, 59.2061) (-7.0536, 59.1202) (-7.0654, 59.0413) (-7.0759, 58.9695) (-7.0855, 58.9031) (-7.0946, 58.8392) (-7.1035, 58.775) (-7.1124, 58.7085) (-7.1217, 58.639) (-7.1314, 58.5666) (-7.1416, 58.4919) (-7.152, 58.4162) (-7.1625, 58.3404) (-7.1727, 58.2657) (-7.1824, 58.1926) (-7.1915, 58.1209) (-7.2002, 58.0493) (-7.2087, 57.9764) (-7.2174, 57.9005) (-7.2265, 57.8206) (-7.2359, 57.7364) (-7.2456, 57.6486) (-7.2552, 57.5584) (-7.2646, 57.4672) (-7.2736, 57.3769) (-7.2821, 57.2889) (-7.2901, 57.2046) (-7.2977, 57.1248) (-7.3048, 57.0496) (-7.3115, 56.9782) (-7.318, 56.9088) (-7.3244, 56.8391) (-7.3307, 56.7658) (-7.3372, 56.6856) (-7.3442, 56.5945) (-7.3518, 56.4891) (-7.3603, 56.3661) (-7.3699, 56.2229) (-7.3806, 56.0582) (-7.3925, 55.8718) (-7.4053, 55.6647) (-7.4189, 55.4387) (-7.433, 55.1966) (-7.4474, 54.9415) (-7.4617, 54.677) (-7.4756, 54.4069) (-7.4888, 54.1352) (-7.5011, 53.8654) (-7.5122, 53.6012) (-7.522, 53.3455) (-7.5305, 53.1006) (-7.5377, 52.8683) (-7.5436, 52.6498) (-7.5484, 52.4457) (-7.5522, 52.2561) (-7.5552, 52.0807) (-7.5576, 51.9186) (-7.5595, 51.7685) (-7.5611, 51.6286) (-7.5624, 51.4967) (-7.5636, 51.3702) (-7.5646, 51.2466) (-7.5654, 51.1229) (-7.5661, 50.9966) (-7.5666, 50.8653) (-7.5669, 50.7268) (-7.567, 50.5796) (-7.5669, 50.4226) (-7.5665, 50.2548) (-7.5659, 50.0757) (-7.5651, 49.8851) (-7.5642, 49.7231) (-7.5634, 49.5963) (-7.5628, 49.5094) (-7.5625, 49.4653) knots 0 0 0 0 0 0 0.00689655 0.0137931 0.02068966 0.02758621 0.03448276 0.04137931 0.04827586 0.05517241 0.06206897 0.06896552 0.07586207 0.08275862 0.08965517 0.09655172 0.10344828 0.11034483 0.11724138 0.12413793 0.13103448 0.13793103 0.14482759 0.15172414 0.15862069 0.16551724 0.17241379 0.17931034 0.1862069 0.19310345 0.2 0.20689655 0.2137931 0.22068966 0.22758621 0.23448276 0.24137931 0.24827586 0.25517241 0.26206897 0.26896552 0.27586207 0.28275862 0.28965517 0.29655172 0.30344828 0.31034483 0.31724138 0.32413793 0.33103448 0.33793103 0.34482759 0.35172414 0.35862069 0.36551724 0.37241379 0.37931034 0.3862069 0.39310345 0.4 0.40689655 0.4137931 0.42068966 0.42758621 0.43448276 0.44137931 0.44827586 0.45517241 0.46206897 0.46896552 0.47586207 0.48275862 0.48965517 0.49655172 0.50344828 0.51034483 0.51724138 0.52413793 0.53103448 0.53793103 0.54482759 0.55172414 0.55862069 0.56551724 0.57241379 0.57931034 0.5862069 0.59310345 0.6 0.60689655 0.6137931 0.62068966 0.62758621 0.63448276 0.64137931 0.64827586 0.65517241 0.66206897 0.66896552 0.67586207 0.68275862 0.68965517 0.69655172 0.70344828 0.71034483 0.71724138 0.72413793 0.73103448 0.73793103 0.74482759 0.75172414 0.75862069 0.76551724 0.77241379 0.77931034 0.7862069 0.79310345 0.8 0.80689655 0.8137931 0.82068966 0.82758621 0.83448276 0.84137931 0.84827586 0.85517241 0.86206897 0.86896552 0.87586207 0.88275862 0.88965517 0.89655172 0.90344828 0.91034483 0.91724138 0.92413793 0.93103448 0.93793103 0.94482759 0.95172414 0.95862069 0.96551724 0.97241379 0.97931034 0.9862069 0.99310345 1 1 1 1 1 1
  spline S1 degree 5 poles (-7.5625, 49.4653) (-7.5655, 49.3307) (-7.57, 49.0496) (-7.572, 48.5928) (-7.5661, 47.9124) (-7.5379, 46.9635) (-7.4825, 45.9635) (-7.3594, 45.0422) (-7.344, 44.226) (-7.6467, 43.4795) (-8.3052, 42.6439) (-9.1392, 41.6182) (-10.0385, 40.5852) (-10.8877, 39.7191) (-11.6091, 39.1406) (-12.1643, 38.5973) (-12.5444, 37.8768) (-12.7555, 36.8923) (-12.8172, 35.6021) (-12.7558, 33.9978) (-12.602, 32.0799) (-12.389, 29.8619) (-12.151, 27.3636) (-11.9215, 24.6101) (-11.732, 21.6278) (-11.61, 18.4421) (-11.5838, 15.7481) (-11.6109, 13.6525) (-11.6505, 12.2229) (-11.6757, 11.5) knots 0 0 0 0 0 0 0.04 0.08 0.12 0.16 0.2 0.24 0.28 0.32 0.36 0.4 0.44 0.48 0.52 0.56 0.6 0.64 0.68 0.72 0.76 0.8 0.84 0.88 0.92 0.96 1 1 1 1 1 1
  spline S2 degree 5 poles (-11.6757, 11.5) (-11.6505, 10.7771) (-11.6109, 9.3475) (-11.5838, 7.2519) (-11.61, 4.5579) (-11.732, 1.3722) (-11.9215, -1.6101) (-12.151, -4.3636) (-12.389, -6.8619) (-12.602, -9.0799) (-12.7558, -10.9978) (-12.8172, -12.6021) (-12.7555, -13.8923) (-12.5444, -14.8768) (-12.1643, -15.5973) (-11.6091, -16.1406) (-10.8877, -16.7191) (-10.0385, -17.5852) (-9.1392, -18.6182) (-8.3052, -19.6439) (-7.6467, -20.4795) (-7.344, -21.226) (-7.3594, -22.0422) (-7.4825, -22.9635) (-7.5379, -23.9635) (-7.5661, -24.9124) (-7.572, -25.5928) (-7.57, -26.0496) (-7.5655, -26.3307) (-7.5625, -26.4653) knots -1 -1 -1 -1 -1 -1 -0.96 -0.92 -0.88 -0.84 -0.8 -0.76 -0.72 -0.68 -0.64 -0.6 -0.56 -0.52 -0.48 -0.44 -0.4 -0.36 -0.32 -0.28 -0.24 -0.2 -0.16 -0.12 -0.08 -0.04 0 0 0 0 0 0
  spline S3 degree 5 poles (-7.5625, -26.4653) (-7.5628, -26.5094) (-7.5634, -26.5963) (-7.5642, -26.7231) (-7.5651, -26.8851) (-7.5659, -27.0757) (-7.5665, -27.2548) (-7.5669, -27.4226) (-7.567, -27.5796) (-7.5669, -27.7268) (-7.5666, -27.8653) (-7.5661, -27.9966) (-7.5654, -28.1229) (-7.5646, -28.2466) (-7.5636, -28.3702) (-7.5624, -28.4967) (-7.5611, -28.6286) (-7.5595, -28.7685) (-7.5576, -28.9186) (-7.5552, -29.0807) (-7.5522, -29.2561) (-7.5484, -29.4457) (-7.5436, -29.6498) (-7.5377, -29.8683) (-7.5305, -30.1006) (-7.522, -30.3455) (-7.5122, -30.6012) (-7.5011, -30.8654) (-7.4888, -31.1352) (-7.4756, -31.4069) (-7.4617, -31.677) (-7.4474, -31.9415) (-7.433, -32.1966) (-7.4189, -32.4387) (-7.4053, -32.6647) (-7.3925, -32.8718) (-7.3806, -33.0582) (-7.3699, -33.2229) (-7.3603, -33.3661) (-7.3518, -33.4891) (-7.3442, -33.5945) (-7.3372, -33.6856) (-7.3307, -33.7658) (-7.3244, -33.8391) (-7.318, -33.9088) (-7.3115, -33.9782) (-7.3048, -34.0496) (-7.2977, -34.1248) (-7.2901, -34.2046) (-7.2821, -34.2889) (-7.2736, -34.3769) (-7.2646, -34.4672) (-7.2552, -34.5584) (-7.2456, -34.6486) (-7.2359, -34.7364) (-7.2265, -34.8206) (-7.2174, -34.9005) (-7.2087, -34.9764) (-7.2002, -35.0493) (-7.1915, -35.1209) (-7.1824, -35.1926) (-7.1727, -35.2657) (-7.1625, -35.3404) (-7.152, -35.4162) (-7.1416, -35.4919) (-7.1314, -35.5666) (-7.1217, -35.639) (-7.1124, -35.7085) (-7.1035, -35.775) (-7.0946, -35.8392) (-7.0855, -35.9031) (-7.0759, -35.9695) (-7.0654, -36.0413) (-7.0536, -36.1202) (-7.0406, -36.2061) (-7.0261, -36.2973) (-7.0103, -36.3909) (-6.9934, -36.4839) (-6.9757, -36.5739) (-6.9576, -36.6596) (-6.9395, -36.7407) (-6.922, -36.8176) (-6.9052, -36.8908) (-6.8893, -36.9608) (-6.8743, -37.0273) (-6.8597, -37.0905) (-6.8451, -37.1506) (-6.8302, -37.2087) (-6.8143, -37.2668) (-6.7971, -37.3266) (-6.7786, -37.3886) (-6.7593, -37.4514) (-6.7401, -37.5116) (-6.7216, -37.5664) (-6.7041, -37.6146) (-6.6867, -37.6585) (-6.6682, -37.7019) (-6.6475, -37.7483) (-6.6247, -37.7981) (-6.6006, -37.849) (-6.5761, -37.8985) (-6.5515, -37.9451) (-6.526, -37.9902) (-6.4986, -38.0364) (-6.4682, -38.0857) (-6.4348, -38.1384) (-6.399, -38.1932) (-6.3617, -38.2481) (-6.3238, -38.3017) (-6.2854, -38.3535) (-6.2464, -38.4044) (-6.2058, -38.4556) (-6.1625, -38.5087) (-6.1145, -38.5652) (-6.0602, -38.6264) (-5.9978, -38.693) (-5.9267, -38.765) (-5.847, -38.8412) (-5.7601, -38.9197) (-5.6681, -38.9982) (-5.5733, -39.074) (-5.4785, -39.1451) (-5.3861, -39.2095) (-5.2984, -39.2666) (-5.2168, -39.3165) (-5.1421, -39.3599) (-5.0739, -39.398) (-5.0108, -39.4326) (-4.9498, -39.4653) (-4.887, -39.4978) (-4.8188, -39.5315) (-4.7423, -39.5672) (-4.6561, -39.6046) (-4.5606, -39.6428) (-4.457, -39.6802) (-4.3473, -39.7155) (-4.2334, -39.7472) (-4.1173, -39.7746) (-4.0002, -39.7977) (-3.8833, -39.8166) (-3.7672, -39.8322) (-3.6523, -39.8451) (-3.539, -39.8561) (-3.4274, -39.866) (-3.3178, -39.8751) (-3.2101, -39.8836) (-3.1256, -39.8901) (-3.0631, -39.8948) (-3.0218, -39.8979) (-3.0013, -39.8994) knots -1 -1 -1 -1 -1 -1 -0.99310345 -0.9862069 -0.97931034 -0.97241379 -0.96551724 -0.95862069 -0.95172414 -0.94482759 -0.93793103 -0.93103448 -0.92413793 -0.91724138 -0.91034483 -0.90344828 -0.89655172 -0.88965517 -0.88275862 -0.87586207 -0.86896552 -0.86206897 -0.85517241 -0.84827586 -0.84137931 -0.83448276 -0.82758621 -0.82068966 -0.8137931 -0.80689655 -0.8 -0.79310345 -0.7862069 -0.77931034 -0.77241379 -0.76551724 -0.75862069 -0.75172414 -0.74482759 -0.73793103 -0.73103448 -0.72413793 -0.71724138 -0.71034483 -0.70344828 -0.69655172 -0.68965517 -0.68275862 -0.67586207 -0.66896552 -0.66206897 -0.65517241 -0.64827586 -0.64137931 -0.63448276 -0.62758621 -0.62068966 -0.6137931 -0.60689655 -0.6 -0.59310345 -0.5862069 -0.57931034 -0.57241379 -0.56551724 -0.55862069 -0.55172414 -0.54482759 -0.53793103 -0.53103448 -0.52413793 -0.51724138 -0.51034483 -0.50344828 -0.49655172 -0.48965517 -0.48275862 -0.47586207 -0.46896552 -0.46206897 -0.45517241 -0.44827586 -0.44137931 -0.43448276 -0.42758621 -0.42068966 -0.4137931 -0.40689655 -0.4 -0.39310345 -0.3862069 -0.37931034 -0.37241379 -0.36551724 -0.35862069 -0.35172414 -0.34482759 -0.33793103 -0.33103448 -0.32413793 -0.31724138 -0.31034483 -0.30344828 -0.29655172 -0.28965517 -0.28275862 -0.27586207 -0.26896552 -0.26206897 -0.25517241 -0.24827586 -0.24137931 -0.23448276 -0.22758621 -0.22068966 -0.2137931 -0.20689655 -0.2 -0.19310345 -0.1862069 -0.17931034 -0.17241379 -0.16551724 -0.15862069 -0.15172414 -0.14482759 -0.13793103 -0.13103448 -0.12413793 -0.11724138 -0.11034483 -0.10344828 -0.09655172 -0.08965517 -0.08275862 -0.07586207 -0.06896552 -0.06206897 -0.05517241 -0.04827586 -0.04137931 -0.03448276 -0.02758621 -0.02068966 -0.0137931 -0.00689655 0 0 0 0 0 0
  line L2 (-3.0013, -39.8994) -> (-1.5, -39.8994)
  line L3 (-1.5, -39.8994) -> (0.0013, -39.8994)
  spline S4 degree 5 poles (0.0013, -39.8994) (0.0218, -39.8979) (0.0631, -39.8948) (0.1256, -39.8901) (0.2101, -39.8836) (0.3178, -39.8751) (0.4274, -39.866) (0.539, -39.8561) (0.6523, -39.8451) (0.7672, -39.8322) (0.8833, -39.8166) (1.0002, -39.7977) (1.1173, -39.7746) (1.2334, -39.7472) (1.3473, -39.7155) (1.457, -39.6802) (1.5606, -39.6428) (1.6561, -39.6046) (1.7423, -39.5672) (1.8188, -39.5315) (1.887, -39.4978) (1.9498, -39.4653) (2.0108, -39.4326) (2.0739, -39.398) (2.1421, -39.3599) (2.2168, -39.3165) (2.2984, -39.2666) (2.3861, -39.2095) (2.4785, -39.1451) (2.5733, -39.074) (2.6681, -38.9982) (2.7601, -38.9197) (2.847, -38.8412) (2.9267, -38.765) (2.9978, -38.693) (3.0602, -38.6264) (3.1145, -38.5652) (3.1625, -38.5087) (3.2058, -38.4556) (3.2464, -38.4044) (3.2854, -38.3535) (3.3238, -38.3017) (3.3617, -38.2481) (3.399, -38.1932) (3.4348, -38.1384) (3.4682, -38.0857) (3.4986, -38.0364) (3.526, -37.9902) (3.5515, -37.9451) (3.5761, -37.8985) (3.6006, -37.849) (3.6247, -37.7981) (3.6475, -37.7483) (3.6682, -37.7019) (3.6867, -37.6585) (3.7041, -37.6146) (3.7216, -37.5664) (3.7401, -37.5116) (3.7593, -37.4514) (3.7786, -37.3886) (3.7971, -37.3266) (3.8143, -37.2668) (3.8302, -37.2087) (3.8451, -37.1506) (3.8597, -37.0905) (3.8743, -37.0273) (3.8893, -36.9608) (3.9052, -36.8908) (3.922, -36.8176) (3.9395, -36.7407) (3.9576, -36.6596) (3.9757, -36.5739) (3.9934, -36.4839) (4.0103, -36.3909) (4.0261, -36.2973) (4.0406, -36.2061) (4.0536, -36.1202) (4.0654, -36.0413) (4.0759, -35.9695) (4.0855, -35.9031) (4.0946, -35.8392) (4.1035, -35.775) (4.1124, -35.7085) (4.1217, -35.639) (4.1314, -35.5666) (4.1416, -35.4919) (4.152, -35.4162) (4.1625, -35.3404) (4.1727, -35.2657) (4.1824, -35.1926) (4.1915, -35.1209) (4.2002, -35.0493) (4.2087, -34.9764) (4.2174, -34.9005) (4.2265, -34.8206) (4.2359, -34.7364) (4.2456, -34.6486) (4.2552, -34.5584) (4.2646, -34.4672) (4.2736, -34.3769) (4.2821, -34.2889) (4.2901, -34.2046) (4.2977, -34.1248) (4.3048, -34.0496) (4.3115, -33.9782) (4.318, -33.9088) (4.3244, -33.8391) (4.3307, -33.7658) (4.3372, -33.6856) (4.3442, -33.5945) (4.3518, -33.4891) (4.3603, -33.3661) (4.3699, -33.2229) (4.3806, -33.0582) (4.3925, -32.8718) (4.4053, -32.6647) (4.4189, -32.4387) (4.433, -32.1966) (4.4474, -31.9415) (4.4617, -31.677) (4.4756, -31.4069) (4.4888, -31.1352) (4.5011, -30.8654) (4.5122, -30.6012) (4.522, -30.3455) (4.5305, -30.1006) (4.5377, -29.8683) (4.5436, -29.6498) (4.5484, -29.4457) (4.5522, -29.2561) (4.5552, -29.0807) (4.5576, -28.9186) (4.5595, -28.7685) (4.5611, -28.6286) (4.5624, -28.4967) (4.5636, -28.3702) (4.5646, -28.2466) (4.5654, -28.1229) (4.5661, -27.9966) (4.5666, -27.8653) (4.5669, -27.7268) (4.567, -27.5796) (4.5669, -27.4226) (4.5665, -27.2548) (4.5659, -27.0757) (4.5651, -26.8851) (4.5642, -26.7231) (4.5634, -26.5963) (4.5628, -26.5094) (4.5625, -26.4653) knots 0 0 0 0 0 0 0.00689655 0.0137931 0.02068966 0.02758621 0.03448276 0.04137931 0.04827586 0.05517241 0.06206897 0.06896552 0.07586207 0.08275862 0.08965517 0.09655172 0.10344828 0.11034483 0.11724138 0.12413793 0.13103448 0.13793103 0.14482759 0.15172414 0.15862069 0.16551724 0.17241379 0.17931034 0.1862069 0.19310345 0.2 0.20689655 0.2137931 0.22068966 0.22758621 0.23448276 0.24137931 0.24827586 0.25517241 0.26206897 0.26896552 0.27586207 0.28275862 0.28965517 0.29655172 0.30344828 0.31034483 0.31724138 0.32413793 0.33103448 0.33793103 0.34482759 0.35172414 0.35862069 0.36551724 0.37241379 0.37931034 0.3862069 0.39310345 0.4 0.40689655 0.4137931 0.42068966 0.42758621 0.43448276 0.44137931 0.44827586 0.45517241 0.46206897 0.46896552 0.47586207 0.48275862 0.48965517 0.49655172 0.50344828 0.51034483 0.51724138 0.52413793 0.53103448 0.53793103 0.54482759 0.55172414 0.55862069 0.56551724 0.57241379 0.57931034 0.5862069 0.59310345 0.6 0.60689655 0.6137931 0.62068966 0.62758621 0.63448276 0.64137931 0.64827586 0.65517241 0.66206897 0.66896552 0.67586207 0.68275862 0.68965517 0.69655172 0.70344828 0.71034483 0.71724138 0.72413793 0.73103448 0.73793103 0.74482759 0.75172414 0.75862069 0.76551724 0.77241379 0.77931034 0.7862069 0.79310345 0.8 0.80689655 0.8137931 0.82068966 0.82758621 0.83448276 0.84137931 0.84827586 0.85517241 0.86206897 0.86896552 0.87586207 0.88275862 0.88965517 0.89655172 0.90344828 0.91034483 0.91724138 0.92413793 0.93103448 0.93793103 0.94482759 0.95172414 0.95862069 0.96551724 0.97241379 0.97931034 0.9862069 0.99310345 1 1 1 1 1 1
  spline S5 degree 5 poles (4.5625, -26.4653) (4.5655, -26.3307) (4.57, -26.0496) (4.572, -25.5928) (4.5661, -24.9124) (4.5379, -23.9635) (4.4825, -22.9635) (4.3594, -22.0422) (4.344, -21.226) (4.6467, -20.4795) (5.3052, -19.6439) (6.1392, -18.6182) (7.0385, -17.5852) (7.8877, -16.7191) (8.6091, -16.1406) (9.1643, -15.5973) (9.5444, -14.8768) (9.7555, -13.8923) (9.8172, -12.6021) (9.7558, -10.9978) (9.602, -9.0799) (9.389, -6.8619) (9.151, -4.3636) (8.9215, -1.6101) (8.732, 1.3722) (8.61, 4.5579) (8.5838, 7.2519) (8.6109, 9.3475) (8.6505, 10.7771) (8.6757, 11.5) knots 0 0 0 0 0 0 0.04 0.08 0.12 0.16 0.2 0.24 0.28 0.32 0.36 0.4 0.44 0.48 0.52 0.56 0.6 0.64 0.68 0.72 0.76 0.8 0.84 0.88 0.92 0.96 1 1 1 1 1 1
  spline S6 degree 5 poles (8.6757, 11.5) (8.6505, 12.2229) (8.6109, 13.6525) (8.5838, 15.7481) (8.61, 18.4421) (8.732, 21.6278) (8.9215, 24.6101) (9.151, 27.3636) (9.389, 29.8619) (9.602, 32.0799) (9.7558, 33.9978) (9.8172, 35.6021) (9.7555, 36.8923) (9.5444, 37.8768) (9.1643, 38.5973) (8.6091, 39.1406) (7.8877, 39.7191) (7.0385, 40.5852) (6.1392, 41.6182) (5.3052, 42.6439) (4.6467, 43.4795) (4.344, 44.226) (4.3594, 45.0422) (4.4825, 45.9635) (4.5379, 46.9635) (4.5661, 47.9124) (4.572, 48.5928) (4.57, 49.0496) (4.5655, 49.3307) (4.5625, 49.4653) knots -1 -1 -1 -1 -1 -1 -0.96 -0.92 -0.88 -0.84 -0.8 -0.76 -0.72 -0.68 -0.64 -0.6 -0.56 -0.52 -0.48 -0.44 -0.4 -0.36 -0.32 -0.28 -0.24 -0.2 -0.16 -0.12 -0.08 -0.04 0 0 0 0 0 0
  spline S7 degree 5 poles (4.5625, 49.4653) (4.5628, 49.5094) (4.5634, 49.5963) (4.5642, 49.7231) (4.5651, 49.8851) (4.5659, 50.0757) (4.5665, 50.2548) (4.5669, 50.4226) (4.567, 50.5796) (4.5669, 50.7268) (4.5666, 50.8653) (4.5661, 50.9966) (4.5654, 51.1229) (4.5646, 51.2466) (4.5636, 51.3702) (4.5624, 51.4967) (4.5611, 51.6286) (4.5595, 51.7685) (4.5576, 51.9186) (4.5552, 52.0807) (4.5522, 52.2561) (4.5484, 52.4457) (4.5436, 52.6498) (4.5377, 52.8683) (4.5305, 53.1006) (4.522, 53.3455) (4.5122, 53.6012) (4.5011, 53.8654) (4.4888, 54.1352) (4.4756, 54.4069) (4.4617, 54.677) (4.4474, 54.9415) (4.433, 55.1966) (4.4189, 55.4387) (4.4053, 55.6647) (4.3925, 55.8718) (4.3806, 56.0582) (4.3699, 56.2229) (4.3603, 56.3661) (4.3518, 56.4891) (4.3442, 56.5945) (4.3372, 56.6856) (4.3307, 56.7658) (4.3244, 56.8391) (4.318, 56.9088) (4.3115, 56.9782) (4.3048, 57.0496) (4.2977, 57.1248) (4.2901, 57.2046) (4.2821, 57.2889) (4.2736, 57.3769) (4.2646, 57.4672) (4.2552, 57.5584) (4.2456, 57.6486) (4.2359, 57.7364) (4.2265, 57.8206) (4.2174, 57.9005) (4.2087, 57.9764) (4.2002, 58.0493) (4.1915, 58.1209) (4.1824, 58.1926) (4.1727, 58.2657) (4.1625, 58.3404) (4.152, 58.4162) (4.1416, 58.4919) (4.1314, 58.5666) (4.1217, 58.639) (4.1124, 58.7085) (4.1035, 58.775) (4.0946, 58.8392) (4.0855, 58.9031) (4.0759, 58.9695) (4.0654, 59.0413) (4.0536, 59.1202) (4.0406, 59.2061) (4.0261, 59.2973) (4.0103, 59.3909) (3.9934, 59.4839) (3.9757, 59.5739) (3.9576, 59.6596) (3.9395, 59.7407) (3.922, 59.8176) (3.9052, 59.8908) (3.8893, 59.9608) (3.8743, 60.0273) (3.8597, 60.0905) (3.8451, 60.1506) (3.8302, 60.2087) (3.8143, 60.2668) (3.7971, 60.3266) (3.7786, 60.3886) (3.7593, 60.4514) (3.7401, 60.5116) (3.7216, 60.5664) (3.7041, 60.6146) (3.6867, 60.6585) (3.6682, 60.7019) (3.6475, 60.7483) (3.6247, 60.7981) (3.6006, 60.849) (3.5761, 60.8985) (3.5515, 60.9451) (3.526, 60.9902) (3.4986, 61.0364) (3.4682, 61.0857) (3.4348, 61.1384) (3.399, 61.1932) (3.3617, 61.2481) (3.3238, 61.3017) (3.2854, 61.3535) (3.2464, 61.4044) (3.2058, 61.4556) (3.1625, 61.5087) (3.1145, 61.5652) (3.0602, 61.6264) (2.9978, 61.693) (2.9267, 61.765) (2.847, 61.8412) (2.7601, 61.9197) (2.6681, 61.9982) (2.5733, 62.074) (2.4785, 62.1451) (2.3861, 62.2095) (2.2984, 62.2666) (2.2168, 62.3165) (2.1421, 62.3599) (2.0739, 62.398) (2.0108, 62.4326) (1.9498, 62.4653) (1.887, 62.4978) (1.8188, 62.5315) (1.7423, 62.5672) (1.6561, 62.6046) (1.5606, 62.6428) (1.457, 62.6802) (1.3473, 62.7155) (1.2334, 62.7472) (1.1173, 62.7746) (1.0002, 62.7977) (0.8833, 62.8166) (0.7672, 62.8322) (0.6523, 62.8451) (0.539, 62.8561) (0.4274, 62.866) (0.3178, 62.8751) (0.2101, 62.8836) (0.1256, 62.8901) (0.0631, 62.8948) (0.0218, 62.8979) (0.0013, 62.8994) knots -1 -1 -1 -1 -1 -1 -0.99310345 -0.9862069 -0.97931034 -0.97241379 -0.96551724 -0.95862069 -0.95172414 -0.94482759 -0.93793103 -0.93103448 -0.92413793 -0.91724138 -0.91034483 -0.90344828 -0.89655172 -0.88965517 -0.88275862 -0.87586207 -0.86896552 -0.86206897 -0.85517241 -0.84827586 -0.84137931 -0.83448276 -0.82758621 -0.82068966 -0.8137931 -0.80689655 -0.8 -0.79310345 -0.7862069 -0.77931034 -0.77241379 -0.76551724 -0.75862069 -0.75172414 -0.74482759 -0.73793103 -0.73103448 -0.72413793 -0.71724138 -0.71034483 -0.70344828 -0.69655172 -0.68965517 -0.68275862 -0.67586207 -0.66896552 -0.66206897 -0.65517241 -0.64827586 -0.64137931 -0.63448276 -0.62758621 -0.62068966 -0.6137931 -0.60689655 -0.6 -0.59310345 -0.5862069 -0.57931034 -0.57241379 -0.56551724 -0.55862069 -0.55172414 -0.54482759 -0.53793103 -0.53103448 -0.52413793 -0.51724138 -0.51034483 -0.50344828 -0.49655172 -0.48965517 -0.48275862 -0.47586207 -0.46896552 -0.46206897 -0.45517241 -0.44827586 -0.44137931 -0.43448276 -0.42758621 -0.42068966 -0.4137931 -0.40689655 -0.4 -0.39310345 -0.3862069 -0.37931034 -0.37241379 -0.36551724 -0.35862069 -0.35172414 -0.34482759 -0.33793103 -0.33103448 -0.32413793 -0.31724138 -0.31034483 -0.30344828 -0.29655172 -0.28965517 -0.28275862 -0.27586207 -0.26896552 -0.26206897 -0.25517241 -0.24827586 -0.24137931 -0.23448276 -0.22758621 -0.22068966 -0.2137931 -0.20689655 -0.2 -0.19310345 -0.1862069 -0.17931034 -0.17241379 -0.16551724 -0.15862069 -0.15172414 -0.14482759 -0.13793103 -0.13103448 -0.12413793 -0.11724138 -0.11034483 -0.10344828 -0.09655172 -0.08965517 -0.08275862 -0.07586207 -0.06896552 -0.06206897 -0.05517241 -0.04827586 -0.04137931 -0.03448276 -0.02758621 -0.02068966 -0.0137931 -0.00689655 0 0 0 0 0 0
  line L4 (10, 11.5) -> (-13, 11.5)
  line L5 (-1.5, 63) -> (-1.5, -40)
  line L6 (4.5335, -30) -> (-7.5335, -30)
  line L7 (4.5335, 53) -> (-7.5335, 53)
hidden bodies 1
